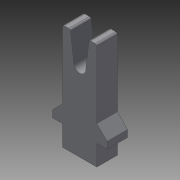
# Autodesk Inventor part: arm 1
Saved by Autodesk Inventor 2015 (Build 190159000, 159)
## iProperties
Created: 2015-06-16
Part Number: arm 1
Material: Generic
Document SubType Name: Modeling
Designer: Robert Allen Fett
Density: 1 g/cm^3
Appearance: Default
Author: Robert Allen Fett
Autodesk Inventor part; units mm, degrees
ref_plane "YZ Plane" through (0, 0, 0) normal (1, 0, 0) x (0, 1, 0)
ref_plane "XZ Plane" through (0, 0, 0) normal (0, 1, 0) x (-1, 0, 0)
ref_plane "XY Plane" through (0, 0, 0) normal (0, 0, 1) x (1, 0, 0)
sketch "Sketch1" plane through (0, 0, 0) normal (0, 0, 1) x (1, 0, 0)
  line L0 (0, -6) -> (0, 0) projected
  line L1 (-9, 0) -> (0, 0) projected
  line L2 (0, -6) -> (-9, -6) projected
  line L3 (0, 0) -> (10, 0) projected
  line L4 (0, 0) -> (0, -6) projected
  line L5 (10, -6) -> (0, -6) projected
  line L6 (10, 0) -> (10, -6) projected
  line L7 (0, -6) -> (-9, -6) projected
  line L8 (-9, 0) -> (0, 0) projected
  line L9 (0, -6) -> (10, -6)
  line L10 (10, -6) -> (10, 0)
  line L11 (10, 0) -> (0, 0)
  line L12 (0, 0) -> (0, -6)
  line L13 (-3, 0) -> (13, 0)
  line L14 (13, 0) -> (13, 2)
  line L15 (13, 2) -> (-3, 2)
  line L16 (-3, 2) -> (-3, 0)
  line L17 (-9, -6) -> (-9, 0) projected
  line L18 (-9, -6) -> (-9, 0) projected
  line L19 (0, -6) -> (0, 0) projected
  point P0 (5, 2)
  point P1 (5, 0)
  dimension "d0" = 16
  dimension "d2" = 2
  constraints: 16 end point, 4 parallel, 2 horizontal, 2 midpoint, 2 perpendicular, 1 point on line, 1 vertical alignment
  measures "d0" distance between parallel lines of L14 L16
  measures "d2" distance of L13.end L14.end
extrude "Extrusion1" add sketch "Sketch1" along normal blind 6 contours L0 L3 L6 L5 | L1 L16 L15 L14 L13 L3
sketch "Sketch2" plane through (0, 0, 6) normal (0, 0, 1) x (1, 0, 0)
  line L0 (0, 0) -> (0, -6) projected
  line L1 (0, -6) -> (10, -6) projected
  line L2 (10, -6) -> (10, 0) projected
  line L3 (13, 2) -> (-3, 2) projected
  line L4 (0, 2) -> (10, 2)
  line L5 (10, 2) -> (10, 25)
  line L6 (10, 25) -> (0, 25)
  line L7 (0, 25) -> (0, 2)
  dimension "d6" = 31
  dimension "d21" = 10
  constraints: 8 end point, 2 collinear, 2 parallel, 1 horizontal, 1 perpendicular, 1 point on line
  measures "d6" distance between parallel lines of L1 L6
  measures "d21" distance between parallel lines of L5 L7
extrude "Extrusion2" add sketch "Sketch2" against normal blind 6
chamfer "Chamfer1" distance 3 angle 45 2 edges at (0, 2, 3) (10, 2, 3)
sketch "Sketch3" plane through (0, 0, 6) normal (0, 0, 1) x (1, 0, 0)
  line L0 (10, 5) -> (10, 25) projected
  line L1 (10, 25) -> (0, 25) projected
  line L2 (0, 25) -> (0, 5) projected
  line L3 (2.25, 25) -> (7.75, 25)
  line L4 (7.75, 25) -> (7.75, 17) construction
  line L5 (7.75, 17) -> (2.25, 17) construction
  line L6 (2.25, 17) -> (2.25, 25) construction
  circle A0 centre (5, 17) radius 1.75
  line L7 (-3, 0) -> (0, 0) projected
  line L8 (0, 0) -> (0, -6) projected
  line L9 (0, -6) -> (10, -6) projected
  line L10 (10, -6) -> (10, 0) projected
  line L11 (10, 0) -> (13, 0) projected
  line L12 (13, 0) -> (13, 2) projected
  line L13 (10, 5) -> (13, 2) projected
  line L14 (10, 5) -> (10, 25) projected
  line L15 (10, 25) -> (0, 25) projected
  line L16 (0, 25) -> (0, 5) projected
  line L17 (-3, 2) -> (0, 5) projected
  line L18 (-3, 2) -> (-3, 0) projected
  line L19 (6.7368, 16.7858) -> (7.75, 25)
  line L20 (2.25, 25) -> (3.2632, 16.7858)
  dimension "d12" = 2.25
  dimension "d13" = 2.25
  dimension "d14" = 8
  dimension "d17" = 3.5
  constraints: 12 end point, 2 parallel, 2 point on circle, 2 point on line, 2 tangent, 1 centre point, 1 horizontal, 1 midpoint, 1 perpendicular
  measures "d12" distance between parallel lines of L6 L2
  measures "d13" distance between parallel lines of L0 L4
  measures "d14" distance between parallel lines of L5 L1
  measures "d17" diameter of A0
extrude "Extrusion3" cut sketch "Sketch3" against normal blind 6 contours L19 A0 L20 L1 | A0
fillet "Fillet1" radius 0.5 4 edges at (7.75, 25, 3) (2.25, 25, 3) (0, 25, 3) (10, 25, 3)
body "Solid1"
